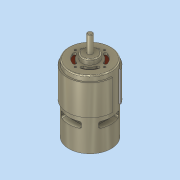
# Autodesk Inventor part: 775-dc-motor
Saved by Autodesk Inventor 2021 (Build 250183000, 183)
## iProperties
Created: 2019-10-15
Part Number: 775-dc-motor
Material: Типовые
Document SubType Name: Modeling
Designer: VADZIM
Density: 1 g/cm^3
Appearance: По умолчанию
Author: VADZIM
Autodesk Inventor part; units mm, degrees
sketch "Sketch1" plane through (0, 0, 0) normal (0, 1, 0) x (-1, 0, 0)
  circle A0 centre (0, 0) radius 21
  dimension "d0" = 42
  constraints: 1 centre point, 1 coincident
  measures "d0" diameter of A0
extrude "Выдавливание1" add sketch "Sketch1" along normal blind 67
ref_plane "РабПлоскость1" through (0, 62, 0) normal (0, 1, 0) x (1, 0, 0)
sketch "Sketch2" plane through (0, 62, 0) normal (0, 1, 0) x (1, 0, 0)
  circle A0 centre (0, 0) radius 22.5
  dimension "d4" = 45
  constraints: 1 centre point, 1 coincident
  measures "d4" diameter of A0
extrude "Выдавливание2" add sketch "Sketch2" against normal blind 30
sketch "Эскиз4" plane through (0, 67, 0) normal (0, 1, 0) x (1, 0, 0)
  circle A0 centre (0, 0) radius 8
  dimension "d7" = 16
  constraints: 1 centre point, 1 coincident
  measures "d7" diameter of A0
extrude "Выдавливание3" add sketch "Эскиз4" along normal blind 5
ref_plane "РабПлоскость2" through (0, 0, -21) normal (0, 0, 1) x (1, 0, 0)
sketch "Эскиз5" plane through (0, 0, -21) normal (0, 0, 1) x (1, 0, 0)
  line L0 (8.5, 27) -> (-8.5, 27)
  line L1 (-10, 25.5) -> (-10, 22.5)
  line L2 (-8.5, 21) -> (8.5, 21)
  line L3 (10, 22.5) -> (10, 25.5)
  line L4 (-22.5, 32) -> (22.5, 32) projected
  arc A0 (8.5, 21) -> (10, 22.5) centre (8.5, 22.5) ccw
  arc A1 (10, 25.5) -> (8.5, 27) centre (8.5, 25.5) ccw
  arc A2 (-8.5, 27) -> (-10, 25.5) centre (-8.5, 25.5) ccw
  arc A3 (-10, 22.5) -> (-8.5, 21) centre (-8.5, 22.5) ccw
  point P0 (0, 0)
  point P1 (-10, 21)
  point P2 (-10, 27)
  point P3 (10, 21)
  point P4 (0, 27)
  dimension "d10" = 5
  dimension "d11" = 6
  dimension "d12" = 20
  dimension "d13" = 1.5
  constraints: 8 end point, 8 point on circle, 8 tangent, 6 point on line, 4 centre point, 3 equal radius, 2 parallel, 1 horizontal, 1 midpoint, 1 perpendicular, 1 vertical alignment
  measures "d10" distance between parallel lines of L4 L0
  measures "d11" distance of point (-10, 27) point (-10, 21)
  measures "d12" distance of point (-10, 21) point (10, 21)
  measures "d13" radius of A0
extrude "Выдавливание4" cut sketch "Эскиз5" along normal blind 6
pattern_circular "Круговой массив1" count 4 over 360 about axis through (0, 72, 0) along (0, 1, 0) of "Выдавливание4"
sketch "Эскиз8" plane through (0, 72, 0) normal (0, 1, 0) x (1, 0, 0)
  circle A0 centre (0, 0) radius 2.5
  dimension "d25" = 5
  constraints: 1 centre point, 1 coincident
  measures "d25" diameter of A0
extrude "Выдавливание7" add sketch "Эскиз8" along normal blind 17
sketch "Эскиз9" plane through (0, 0, 0) normal (0, -1, 0) x (1, 0, 0)
  circle A0 centre (0, 0) radius 22.5 projected
  circle A1 centre (0, 0) radius 20.5
  dimension "d28" = 41
  constraints: 1 centre point, 1 coincident
  measures "d28" diameter of A1
extrude "Выдавливание8" cut sketch "Эскиз9" against normal blind 3 contours A1
sketch "Эскиз10" plane through (0, 3, 0) normal (0, -1, 0) x (1, 0, 0)
  circle A0 centre (0, 0) radius 6
  dimension "d31" = 12
  constraints: 1 centre point, 1 coincident
  measures "d31" diameter of A0
extrude "Выдавливание9" add sketch "Эскиз10" along normal blind 6
sketch "Эскиз11" plane through (0, -3, 0) normal (0, -1, 0) x (1, 0, 0)
  circle A0 centre (0, 0) radius 2.5
  dimension "d34" = 5
  constraints: 1 centre point, 1 coincident
  measures "d34" diameter of A0
extrude "Выдавливание10" add sketch "Эскиз11" along normal blind 6
sketch "Эскиз12" plane through (0, 3, 0) normal (0, -1, 0) x (1, 0, 0)
  arc A0 (3.2492, -10) -> (10, -3.2492) centre (0, 0) ccw
  line L0 (0, 0) -> (10, -3.2492) construction
  line L1 (0, 0) -> (10.5146, 0) construction
  line L2 (0, 0) -> (3.2492, -10) construction
  arc A1 (4.224, -13) -> (13, -4.224) centre (0, 0) ccw
  arc A2 (3.2492, -10) -> (4.224, -13) centre (3.7366, -11.5) ccw
  arc A3 (13, -4.224) -> (10, -3.2492) centre (11.5, -3.7366) ccw
  dimension "d37" = 18
  dimension "d38" = 54
  constraints: 8 point on circle, 6 end point, 4 centre point, 4 tangent, 1 coincident, 1 equal length, 1 horizontal
  measures "d37" angle of L0 L1
  measures "d38" angle of L2 L0
extrude "Выдавливание11" cut sketch "Эскиз12" against normal blind 6
pattern_circular "Круговой массив2" count 4 over 360 about axis through (0, 72, 0) along (0, 1, 0) of "Выдавливание11"
fillet "Сопряжение1" radius 1.5 1 edges at (-6, -3, 0)
fillet "Сопряжение2" radius 1 2 edges at (-8, 72, 0) (21, 67, 0)
fillet "Сопряжение3" radius 0.5 1 edges at (-2.5, 89, 0)
fillet "Сопряжение4" radius 0.5 1 edges at (-2.5, -9, 0)
ref_plane "РабПлоскость3" through (0, 72, 0) normal (0, 0, -1) x (0, 1, 0)
sketch "Sketch14" plane through (0, 67, 0) normal (0, 1, 0) x (1, 0, 0)
  circle A0 centre (0, 0) radius 20 projected
  line L0 (0, 0) -> (-14.5, 0)
  circle A1 centre (-14.5, 0) radius 1
  line L1 (0, 0) -> (14.5, 0)
  line L2 (15, -8.5) -> (15, 8.5) projected
  circle A2 centre (14.5, 0) radius 1
  line L3 (0, 0) -> (0, -14.5)
  circle A3 centre (0, -14.5) radius 1
  line L4 (0, 0) -> (0, 14.5)
  circle A4 centre (0, 14.5) radius 1
  arc A5 (-4.224, 13) -> (-13, 4.224) centre (0, 0) ccw projected
  arc A6 (-3.2492, 10) -> (-4.224, 13) centre (-3.7366, 11.5) ccw projected
  arc A7 (-3.2492, 10) -> (-10, 3.2492) centre (0, 0) ccw projected
  arc A8 (-13, 4.224) -> (-10, 3.2492) centre (-11.5, 3.7366) ccw projected
  arc A9 (4.224, 13) -> (3.2492, 10) centre (3.7366, 11.5) ccw projected
  arc A10 (13, 4.224) -> (4.224, 13) centre (0, 0) ccw projected
  arc A11 (10, 3.2492) -> (3.2492, 10) centre (0, 0) ccw projected
  arc A12 (10, 3.2492) -> (13, 4.224) centre (11.5, 3.7366) ccw projected
  arc A13 (3.2492, -10) -> (10, -3.2492) centre (0, 0) ccw projected
  arc A14 (13, -4.224) -> (10, -3.2492) centre (11.5, -3.7366) ccw projected
  arc A15 (4.224, -13) -> (13, -4.224) centre (0, 0) ccw projected
  arc A16 (3.2492, -10) -> (4.224, -13) centre (3.7366, -11.5) ccw projected
  arc A17 (-10, -3.2492) -> (-3.2492, -10) centre (0, 0) ccw projected
  arc A18 (-4.224, -13) -> (-3.2492, -10) centre (-3.7366, -11.5) ccw projected
  arc A19 (-13, -4.224) -> (-4.224, -13) centre (0, 0) ccw projected
  arc A20 (-10, -3.2492) -> (-13, -4.224) centre (-11.5, -3.7366) ccw projected
  dimension "d51" = 14.5
  dimension "d52" = 2
  dimension "d53" = 14.5
  dimension "d54" = 2
  dimension "d55" = 14.5
  dimension "d56" = 2
  dimension "d57" = 14.5
  dimension "d58" = 2
  constraints: 8 end point, 4 centre point, 4 coincident, 2 vertical, 1 horizontal, 1 perpendicular
  measures "d51" distance of L0.start L0.end
  measures "d52" diameter of A1
  measures "d53" distance of L0.start L1.end
  measures "d54" diameter of A2
  measures "d55" distance of L0.start L3.end
  measures "d56" diameter of A3
  measures "d57" distance of L0.start L4.end
  measures "d58" diameter of A4
extrude "Extrusion12" cut sketch "Sketch14" against normal blind 2 contours A1 | A2 L2 | A3 | A4 | A2 L2 | A6 A7 A8 A5 | A10 A12 A11 A9 | A13 A14 A15 A16 | A17 A18 A19 A20
thread "Thread1" size "M2x0.4" class "6H" standard "ANSI Metric M Profile" length 9.967
thread "Thread2" size "M2x0.4" class "6H" standard "ANSI Metric M Profile" length 9.967
thread "Thread3" size "M2x0.4" class "6H" standard "ANSI Metric M Profile" length 9.967
thread "Thread4" size "M2x0.4" class "6H" standard "ANSI Metric M Profile" length 9.967
ref_plane "Work Plane4" through (0, 0, 0) normal (0, 0, 1) x (1, 0, 0)
sketch "Sketch15" plane through (0, 0, 0) normal (0, 0, 1) x (1, 0, 0)
  line L0 (22.5, 62) -> (22.5, 32) projected
  line L1 (-22.5, 62) -> (22.5, 62) projected
  line L2 (-22.5, 32) -> (22.5, 32) projected
  line L3 (-21, 32) -> (21, 32) projected
  line L4 (21, 62) -> (21, 32)
  line L5 (0, -28.6) -> (0, 108.6) projected
  point P0 (0, 0)
  constraints: 2 end point, 1 perpendicular, 1 point on line
revolve "Revolution1" cut sketch "Sketch15" angle 30 about axis through (0, -10, 0) along (0, 1, 0) contours L0 L2 L4 L1
